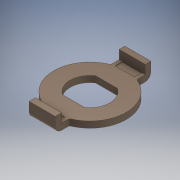
# Autodesk Inventor part: podkładka z dwoma uszami
Saved by Autodesk Inventor 2017 SP1 (Build 210196100, 196)
## iProperties
Created: 2021-02-08
Part Number: podkładka z dwoma uszami
Material: Stal
Document SubType Name: Modeling
Designer: Napoleon
Mass: 0.678015 g
Surface Area: 2.48754 cm^2
Volume: 0.0863713 cm^3
Density: 7.85 g/cm^3
Appearance: Anodowana - ciemnobrązowa
Author: Napoleon
Autodesk Inventor part; units mm, degrees
ref_plane "YZ Plane" through (0, 0, 0) normal (1, 0, 0) x (0, 1, 0)
ref_plane "XZ Plane" through (0, 0, 0) normal (0, 1, 0) x (-1, 0, 0)
ref_plane "XY Plane" through (0, 0, 0) normal (0, 0, 1) x (1, 0, 0)
sketch "Szkic4" plane through (0, 0, 0) normal (0, 0, 1) x (1, 0, 0)
  line L0 (-1.6583, 2.5) -> (1.6583, 2.5)
  line L1 (-1.6583, -2.5) -> (1.6583, -2.5)
  arc A0 (-1.6583, 2.5) -> (-1.6583, -2.5) centre (0, 0) ccw
  arc A1 (1.6583, -2.5) -> (1.6583, 2.5) centre (0, 0) ccw
  line L2 (-1.975, 7.25) -> (1.975, 7.25)
  line L3 (-1.975, 7.25) -> (-1.975, 5.2749)
  line L4 (1.975, 7.25) -> (1.975, 5.2749)
  arc A2 (1.975, 5.2749) -> (2.1278, 5.0446) centre (2.225, 5.2749) ccw
  arc A3 (-2.1278, 5.0446) -> (-1.975, 5.2749) centre (-2.225, 5.2749) ccw
  line L5 (-1.975, -7.25) -> (1.975, -7.25)
  line L6 (-1.975, -7.25) -> (-1.975, -5.2749)
  line L7 (1.975, -7.25) -> (1.975, -5.2749)
  arc A4 (2.1278, -5.0446) -> (1.975, -5.2749) centre (2.225, -5.2749) ccw
  arc A5 (-1.975, -5.2749) -> (-2.1278, -5.0446) centre (-2.225, -5.2749) ccw
  arc A6 (-2.1278, 5.0446) -> (-2.1278, -5.0446) centre (0, 0) ccw
  arc A7 (2.1278, -5.0446) -> (2.1278, 5.0446) centre (0, 0) ccw
  point P0 (-1.975, 5.1064)
  point P1 (1.975, 5.1064)
  point P2 (-1.975, -5.1064)
  point P3 (1.975, -5.1064)
  dimension "d19" = 3.95
  dimension "d20" = 0.25
  constraints: 16 end point, 16 point on circle, 8 centre point, 4 point on line, 2 coincident, 2 horizontal, 2 tangent, 2 vertical, 1 equal radius
  measures "d19" distance of L2.start L2.end
  measures "d20" radius of A2
extrude "Wyciągnięcie proste4" add sketch "Szkic4" along normal mid plane 0.95
sketch "Szkic5" plane through (0, 0, 0.475) normal (0, 0, 1) x (1, 0, 0)
  line L0 (-1.975, 7.25) -> (1.975, 7.25)
  line L1 (1.975, 7.25) -> (1.975, 6.404)
  line L2 (1.975, 6.404) -> (-1.975, 6.404)
  line L3 (-1.975, 6.404) -> (-1.975, 7.25)
  line L4 (1.975, -7.25) -> (-1.975, -7.25)
  line L5 (-1.975, -7.25) -> (-1.975, -6.3)
  line L6 (-1.975, -6.3) -> (1.975, -6.3)
  line L7 (1.975, -6.3) -> (1.975, -7.25)
  dimension "d23" = 0.95
  constraints: 16 end point, 4 parallel, 2 horizontal, 2 perpendicular
  measures "d23" distance of L4.end L5.end
extrude "Wyciągnięcie proste5" add sketch "Szkic5" along normal blind 1.35
fillet "Zaokrąglenie3" radius 0.95 2 edges at (0, 7.25, -0.475) (0, -7.25, -0.475)
sketch "Szkic6" plane through (0, 0, 0.475) normal (0, 0, 1) x (1, 0, 0)
  line L0 (-1.475, 5.2749) -> (1.475, 5.2749)
  line L1 (1.475, 5.2749) -> (1.475, 6.404)
  line L2 (1.475, 6.404) -> (-1.475, 6.404)
  line L3 (-1.475, 6.404) -> (-1.475, 5.2749)
  line L4 (-1.475, -5.2749) -> (1.475, -5.2749)
  line L5 (1.475, -5.2749) -> (1.475, -6.404)
  line L6 (1.475, -6.404) -> (-1.475, -6.404)
  line L7 (-1.475, -6.404) -> (-1.475, -5.2749)
  constraints: 16 end point, 2 parallel, 1 horizontal, 1 perpendicular
extrude "Wyciągnięcie proste6" cut sketch "Szkic6" against normal blind 0.1
